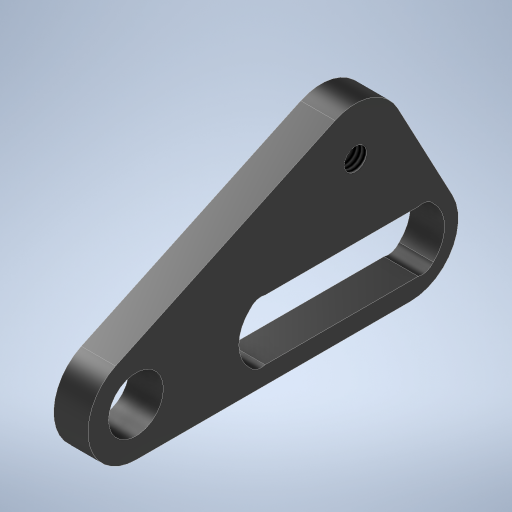
# Autodesk Inventor part: ParallelLinksDriveFrame
Saved by Autodesk Inventor 2024.2 (Build 282272000, 272)
## iProperties
Created: 2024-01-07
Part Number: ParallelLinksDriveFrame
Material: Aluminum 7075
Document SubType Name: Modeling
Designer: Masato Kubotera
Density: 2.81 g/cm^3
Appearance: Glossy - Black
Mass: 11.1082 g
Surface Area: 27.9525 cm^2
Volume: 3.9531 cm^3
Vendor: meviy
Author: Masato Kubotera
Autodesk Inventor part; units mm, degrees
ref_plane "YZ Plane" through (0, 0, 0) normal (1, 0, 0) x (0, 1, 0)
ref_plane "XZ Plane" through (0, 0, 0) normal (0, 1, 0) x (-1, 0, 0)
ref_plane "XY Plane" through (0, 0, 0) normal (0, 0, 1) x (1, 0, 0)
sketch "Sketch1" plane through (0, 0, 0) normal (0, 1, 0) x (-1, 0, 0)
  arc A0 (-2.971, 6.3382) -> (0, -7) centre (0, 0) ccw
  line L0 (0, 0) -> (40, 0) construction
  arc A1 (42.3749, -4.4) -> (42.3749, 4.4) centre (40, 0) ccw
  circle A2 centre (20, 0) radius 20 construction
  circle A3 centre (0, 0) radius 40 construction
  line L1 (42.3749, 4.4) -> (17.6251, 4.4)
  line L2 (0, 0) -> (10, -17.3205) construction
  line L3 (10, -17.3205) -> (20, -34.641) construction
  arc A4 (17.6251, 4.4) -> (17.6251, -4.4) centre (20, 0) ccw
  line L4 (42.3749, -4.4) -> (17.6251, -4.4)
  line L5 (30, 4.4) -> (30, -4.4) construction
  circle A5 centre (40, 0) radius 7 construction
  circle A6 centre (0, 0) radius 7 construction
  circle A7 centre (32, 15) radius 7 construction
  line L6 (-2.971, 6.3382) -> (29.029, 21.3382)
  line L7 (38.1765, 18.2941) -> (46.1765, 3.2941)
  line L8 (0, -7) -> (40, -7)
  arc A8 (40, -7) -> (46.1765, 3.2941) centre (40, 0) ccw
  arc A9 (38.1765, 18.2941) -> (29.029, 21.3382) centre (32, 15) ccw
  arc A10 (43.3651, 3.6981) -> (41.1611, 4.4) centre (41.768, 2.4943) ccw
  arc A11 (41.1611, -4.4) -> (43.3651, -3.6981) centre (41.768, -2.4943) ccw
  arc A12 (18.8389, 4.4) -> (16.6349, 3.6981) centre (18.232, 2.4943) ccw
  arc A13 (16.6349, -3.6981) -> (18.8389, -4.4) centre (18.232, -2.4943) ccw
  circle A14 centre (0, 0) radius 4 construction
  point P0 (16.6349, -3.6981)
  point P1 (16.6349, 3.6981)
  point P2 (18.8389, 4.4)
  point P3 (43.3651, -3.6981)
  point P4 (41.1611, -4.4)
  point P5 (18.8389, -4.4)
  dimension "d0" = 32
  dimension "d1" = 15
  dimension "d2" = 20
  dimension "d3" = 60
  dimension "d4" = 20
  dimension "d5" = 10
  dimension "d6" = 8.8
  dimension "d7" = 20
  dimension "d9" = 14
  dimension "d10" = 2
  dimension "d20" = 8
  constraints: 29 point on circle, 18 end point, 15 centre point, 11 symmetric about line, 10 coincident, 7 tangent, 4 midpoint, 2 equal radius, 2 horizontal, 2 point on line, 1 collinear, 1 parallel, 4 other
  measures "d0" horizontal distance of point (32, 15) A2.start
  measures "d1" vertical distance of point (32, 15) A2.start
  measures "d2" radius of A2
  measures "d3" angle of L2 L0
  measures "d4" distance of L2.end L3.end
  measures "d5" diameter of A1
  measures "d6" distance between parallel lines of L4 L1
  measures "d7" distance of A1.centre A4.centre
  measures "d9" diameter of A6
  measures "d10" radius of A10
  measures "d20" diameter of A14
extrude "Extrusion1" add sketch "Sketch1" along normal blind 5
hole "Phi8.0-h7" at (0, 0, 0) direction (0, 1, 0) diameter 8 end through all
hole "M4" at (-32, 0, 15) direction (0, 1, 0) diameter 3.242 end through all thread size "M4x0.7" class "6H" standard "ANSI Metric M Profile"
equation "\"d7\" = d4"
equation "\"d13\" = d20"
body "Solid1"
